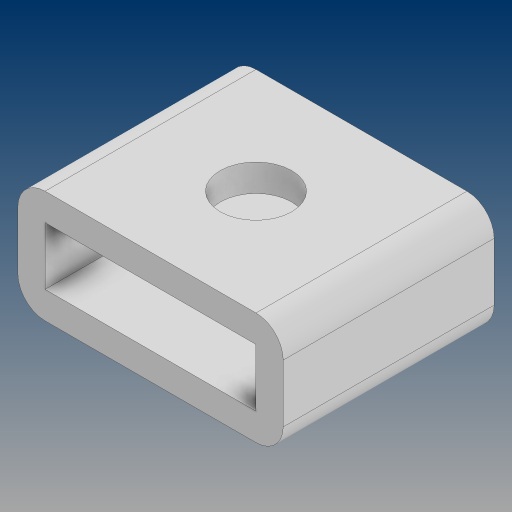
# Autodesk Inventor part: Part3
Saved by Autodesk Inventor 2023 (Build 270158000, 158)
## iProperties
Created: 2023-11-06
Part Number: Part3
Material: Generic
Document SubType Name: Modeling
Designer: gd1
Density: 1 g/cm^3
Appearance: Default
Author: gd1
Autodesk Inventor part; units mm, degrees
ref_plane "YZ Plane" through (0, 0, 0) normal (1, 0, 0) x (0, 1, 0)
ref_plane "XZ Plane" through (0, 0, 0) normal (0, 1, 0) x (-1, 0, 0)
sketch "Sketch1" plane through (0, 0, 0) normal (0, 1, 0) x (-1, 0, 0)
  line L0 (-7.75, -7.75) -> (7.75, -7.75)
  line L1 (7.75, -7.75) -> (7.75, 7.75)
  line L2 (7.75, 7.75) -> (-7.75, 7.75)
  line L3 (-7.75, 7.75) -> (-7.75, -7.75)
  line L4 (-7.75, -7.75) -> (7.75, 7.75) construction
  line L5 (7.75, -7.75) -> (-7.75, 7.75) construction
  line L6 (7.75, 7.75) -> (9.75, 7.75)
  line L7 (9.75, 7.75) -> (9.75, -7.75)
  line L8 (9.75, -7.75) -> (7.75, -7.75)
  line L9 (7.75, -7.75) -> (7.75, 7.75)
  line L10 (-7.75, 7.75) -> (-9.75, 7.75)
  line L11 (-9.75, 7.75) -> (-9.75, -7.75)
  line L12 (-9.75, -7.75) -> (-7.75, -7.75)
  line L13 (-7.75, -7.75) -> (-7.75, 7.75)
  circle A0 centre (0, 0) radius 2.625
  dimension "d0" = 15.5
  dimension "d1" = 15.5
  dimension "d2" = 2
  dimension "d3" = 2
  dimension "d4" = 5.25
  constraints: 28 end point, 6 parallel, 3 horizontal, 3 perpendicular, 2 midpoint, 1 centre point, 1 coincident, 1 point on line
  measures "d0" distance of L2.end L1.end
  measures "d1" distance of L1.end L0.end
  measures "d2" distance of L7.end L8.end
  measures "d3" distance of L12.end L11.end
  measures "d4" diameter of A0
extrude "Extrusion1" add sketch "Sketch1" along normal blind 2 contours L3 L2 L1 L0
extrude "Extrusion2" add sketch "Sketch1" along normal blind 8.25 contours L12 L11 L10 L3 | L1 L6 L7 L8
ref_plane "Work Plane1" through (-9.75, 8.25, 7.75) normal (0, 1, 0) x (1, 0, 0)
sketch "Sketch2" plane through (-9.75, 8.25, 7.75) normal (0, 1, 0) x (1, 0, 0)
  line L0 (0, 0) -> (2, 0) projected
  line L1 (19.5, 15.5) -> (17.5, 15.5) projected
  line L2 (0, 0) -> (19.5, 0)
  line L3 (19.5, 0) -> (19.5, 15.5)
  line L4 (19.5, 15.5) -> (0, 15.5)
  line L5 (0, 15.5) -> (0, 0)
  circle A0 centre (9.75, 7.75) radius 2.625
  line L6 (17.5, 15.5) -> (2, 15.5) projected
  line L7 (0, 0) -> (2, 0)
  line L8 (2, 0) -> (2, 15.5)
  line L9 (2, 15.5) -> (0, 15.5)
  line L10 (0, 15.5) -> (0, 0)
  line L11 (17.5, 0) -> (17.5, 15.5) projected
  line L12 (19.5, 15.5) -> (17.5, 15.5)
  line L13 (17.5, 15.5) -> (17.5, 0)
  line L14 (17.5, 0) -> (19.5, 0)
  line L15 (19.5, 0) -> (19.5, 15.5)
  dimension "d9" = 5.25
  constraints: 24 end point, 6 parallel, 3 horizontal, 3 perpendicular, 1 centre point, 1 coincident
  measures "d9" diameter of A0
extrude "Extrusion3" add sketch "Sketch2" against normal blind 2 contours L8 L4 L11 L2
sketch "Sketch3" plane through (0, 0, 0) normal (0, -1, 0) x (1, 0, 0)
  circle A0 centre (0, 0) radius 7.5
  dimension "d13" = 15
  constraints: 1 centre point, 1 coincident
  measures "d13" diameter of A0
extrude "Extrusion4" cut sketch "Sketch3" against normal blind 0.5
fillet "Fillet2" radius 2 4 edges at (9.75, 8.25, 0) (-9.75, 8.25, 0) (9.75, 0, 0) (-9.75, 0, 0)
body "Solid1"
